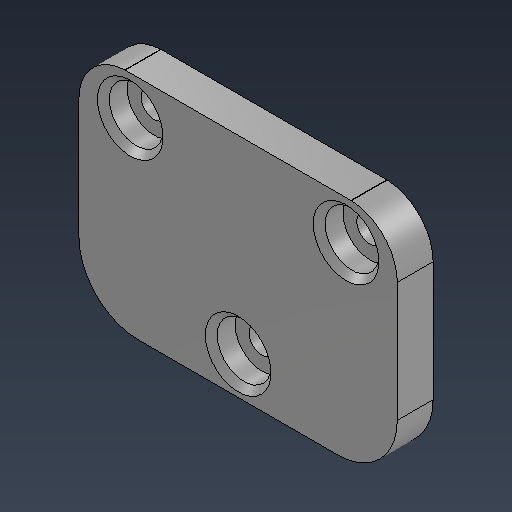
# Autodesk Inventor part: LunasCover
Saved by Autodesk Inventor 2026.2 (Build 302298010, 298A)
## iProperties
Created: 2026-04-20
Part Number: LunasCover
Material: Nylon 6/6
Document SubType Name: Modeling
Designer: szymo
Density: 1.13 g/cm^3
Appearance: Nylon 6(1)
Author: szymo
Autodesk Inventor part; units mm, degrees
ref_plane "YZ Plane" through (0, 0, 0) normal (1, 0, 0) x (0, 1, 0)
ref_plane "XZ Plane" through (0, 0, 0) normal (0, 1, 0) x (-1, 0, 0)
ref_plane "XY Plane" through (0, 0, 0) normal (0, 0, 1) x (1, 0, 0)
sketch "Sketch1" plane through (0, 0, 0) normal (0, 0, 1) x (1, 0, 0)
  circle A0 centre (0.0056, -6.3497) radius 1 projected
  circle A1 centre (-9.0264, 6.2307) radius 1 projected
  circle A2 centre (9.0376, 6.2307) radius 1 projected
  line L0 (9.4418, 9.5) -> (-9.4418, 9.5) projected
  arc A3 (-9.4806, 9.497) -> (-9.4418, 9.5) centre (-9.5, 9.9966) ccw projected
  arc A4 (-9.4806, 9.497) -> (-13.325, 5.5) centre (-9.325, 5.5) ccw projected
  line L1 (-13.325, -4.5) -> (-13.325, 5.5) projected
  arc A5 (-13.325, -4.5) -> (-8.325, -9.5) centre (-8.325, -4.5) ccw projected
  line L2 (8.325, -9.5) -> (-8.325, -9.5) projected
  arc A6 (8.325, -9.5) -> (13.325, -4.5) centre (8.325, -4.5) ccw projected
  line L3 (13.325, 5.5) -> (13.325, -4.5) projected
  arc A7 (13.325, 5.5) -> (9.4806, 9.497) centre (9.325, 5.5) ccw projected
  arc A8 (9.4418, 9.5) -> (9.4806, 9.497) centre (9.5, 9.9966) ccw projected
  point P0 (0, 0)
extrude "Extrusion1" add sketch "Sketch1" along normal blind 3
sketch "Sketch2" plane through (0, 0, 3) normal (0, 0, -1) x (-1, 0, 0)
  circle A0 centre (9.0264, 6.2307) radius 1 projected
  circle A1 centre (-0.0056, -6.3497) radius 1 projected
  circle A2 centre (-9.0376, 6.2307) radius 1 projected
  point P0 (0, 0)
hole "Hole1" at (-9.0264, 6.2307, 3) at (0.0056, -6.3497, 3) at (9.0376, 6.2307, 3) direction (0, 0, -1) diameter 2.2 depth 12 counterbore diameter 4.5 counterbore depth 2 clearance for "Countersunk Flat Head Screw ISO 2009/7046" size "M2" standard "ISO"
chamfer "Chamfer1" distance 0.5 angle 45 3 edges at (-9.0264, 8.4807, 3) (9.0376, 8.4807, 3) (0.0056, -4.0997, 3)
body "Solid1"
